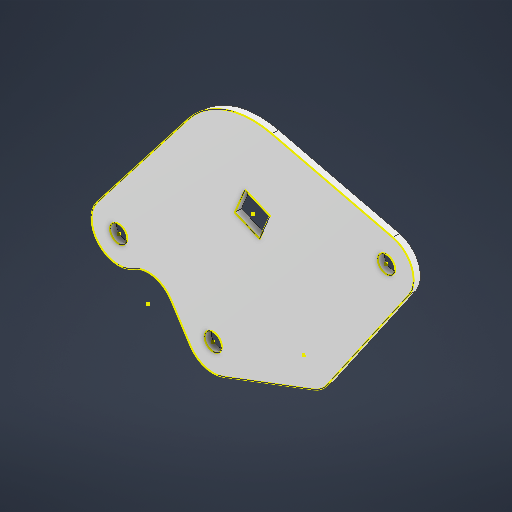
# Autodesk Inventor part: Rear Vertical Odom Pod
Saved by Autodesk Inventor 2025 (Build 290162010, 162A)
## iProperties
Created: 2024-10-31
Part Number: Rear Vertical Odom Pod
Material: Acetal Resin, White
Document SubType Name: Sheet Metal
Designer: blips
Density: 1.425 g/cm^3
Sheet Metal Rule: Default
Appearance: Smooth - White
Author: blips
Autodesk Inventor part; units mm, degrees
ref_plane "YZ Plane" through (0, 0, 0) normal (1, 0, 0) x (0, 1, 0)
ref_plane "XZ Plane" through (0, 0, 0) normal (0, 1, 0) x (-1, 0, 0)
ref_plane "XY Plane" through (0, 0, 0) normal (0, 0, 1) x (1, 0, 0)
sketch "Sketch1" plane through (0, 0, 0) normal (0, 0, 1) x (1, 0, 0)
  circle A0 centre (0, 0) radius 2.0955 construction
  circle A1 centre (31.2825, 19.6012) radius 7.2 construction
  circle A2 centre (43.3748, -2.7357) radius 2.15 construction
  circle A3 centre (31.2825, 19.6012) radius 31.75 construction
  circle A4 centre (43.3748, -2.7357) radius 2.032 construction
  line L0 (31.2825, 19.6012) -> (31.2825, -12.1488) construction
  circle A5 centre (31.2825, -12.1488) radius 2.032 construction
  line L1 (31.2825, 19.6012) -> (62.5502, 25.1146) construction
  line L2 (31.2825, 19.6012) -> (63.0325, 19.6012) construction
  circle A6 centre (62.5502, 25.1146) radius 2.032
  arc A7 (67.7804, 21.5135) -> (64.041, 31.2871) centre (62.5502, 25.1146) ccw
  circle A8 centre (0, 0) radius 2.032
  arc A9 (-5.017, 3.8926) -> (3.4439, -5.335) centre (0, 0) ccw
  arc A10 (45.62, -8.6755) -> (48.605, -6.3367) centre (43.3748, -2.7357) ccw
  circle A11 centre (22.0786, -10.7854) radius 2.032
  line L3 (48.605, -6.3367) -> (67.7804, 21.5135)
  arc A12 (35.755, 38.1188) -> (16.2316, 31.279) centre (31.2825, 19.6012) ccw
  line L4 (64.041, 31.2871) -> (35.755, 38.1188)
  line L5 (-5.017, 3.8926) -> (16.2316, 31.279)
  arc A13 (16.7437, -14.2294) -> (24.3239, -16.7253) centre (22.0786, -10.7854) ccw
  arc A14 (12.2228, -7.226) -> (3.4439, -5.335) centre (6.8878, -10.67) ccw
  line L6 (16.7437, -14.2294) -> (12.2228, -7.226)
  line L7 (45.9985, -8.5324) -> (24.3239, -16.7253)
  line L8 (27.7013, 17.6318) -> (32.3477, 15.7072)
  line L9 (27.7013, 17.6318) -> (27.7013, 17.6318)
  line L10 (32.3477, 15.7072) -> (27.7013, 17.6318)
  line L11 (32.3477, 15.7072) -> (32.3477, 15.7072)
  line L12 (33.1773, 16.0509) -> (35.1019, 20.6973)
  line L13 (33.1773, 16.0509) -> (33.1773, 16.0509)
  line L14 (35.1019, 20.6973) -> (33.1773, 16.0509)
  line L15 (35.1019, 20.6973) -> (35.1019, 20.6973)
  line L16 (34.7583, 21.5269) -> (30.1119, 23.4515)
  line L17 (34.7583, 21.5269) -> (34.7583, 21.5269)
  line L18 (30.1119, 23.4515) -> (34.7583, 21.5269)
  line L19 (30.1119, 23.4515) -> (30.1119, 23.4515)
  line L20 (29.2822, 23.1079) -> (27.3576, 18.4615)
  line L21 (29.2822, 23.1079) -> (29.2822, 23.1079)
  line L22 (27.3576, 18.4615) -> (29.2822, 23.1079)
  line L23 (27.3576, 18.4615) -> (27.3576, 18.4615)
  line L24 (35.1019, 20.6973) -> (35.3449, 21.2839)
  line L25 (34.7583, 21.5269) -> (35.3449, 21.2839)
  line L26 (33.1773, 16.0509) -> (32.9343, 15.4642)
  line L27 (32.3477, 15.7072) -> (32.9343, 15.4642)
  line L28 (29.2822, 23.1079) -> (29.5252, 23.6945)
  line L29 (30.1119, 23.4515) -> (29.5252, 23.6945)
  line L30 (27.3576, 18.4615) -> (27.1146, 17.8748)
  line L31 (27.7013, 17.6318) -> (27.1146, 17.8748)
  point P0 (0, 0)
extrude "Plate1" add sketch "Sketch1" along normal blind 1.5875
sketch "Sketch2" plane through (0, 0, 1.5875) normal (0, 0, 1) x (1, 0, 0)
  arc A0 (-5.017, 3.8926) -> (3.4439, -5.335) centre (0, 0) ccw projected
  line L0 (-5.017, 3.8926) -> (16.2316, 31.279) projected
  arc A1 (35.755, 38.1188) -> (16.2316, 31.279) centre (31.2825, 19.6012) ccw projected
  line L1 (35.755, 38.1188) -> (64.041, 31.2871) projected
  arc A2 (67.7804, 21.5135) -> (64.041, 31.2871) centre (62.5502, 25.1146) ccw projected
  line L2 (67.7804, 21.5135) -> (48.605, -6.3367) projected
  arc A3 (45.62, -8.6755) -> (48.605, -6.3367) centre (43.3748, -2.7357) ccw projected
  line L3 (45.62, -8.6755) -> (24.3239, -16.7253) projected
  arc A4 (16.7437, -14.2294) -> (24.3239, -16.7253) centre (22.0786, -10.7854) ccw projected
  line L4 (16.7437, -14.2294) -> (12.2228, -7.226) projected
  arc A5 (12.2228, -7.226) -> (3.4439, -5.335) centre (6.8878, -10.67) ccw projected
  circle A6 centre (0, 0) radius 2.032 projected
  circle A7 centre (22.0786, -10.7854) radius 2.032 projected
  circle A8 centre (62.5502, 25.1146) radius 2.032 projected
  line L5 (29.5252, 23.6945) -> (35.3449, 21.2839) projected
  line L6 (27.1146, 17.8748) -> (29.5252, 23.6945) projected
  line L7 (35.3449, 21.2839) -> (32.9343, 15.4642) projected
  line L8 (32.9343, 15.4642) -> (27.1146, 17.8748) projected
  point P0 (0, 0)
equation "\"d20\" = Thickness"
equation "\"BendRadius\" = Thickness"
equation "\"BendReliefWidth\" = Thickness"
equation "\"BendReliefDepth\" = 0.5 * Thickness"
equation "\"CornerReliefSize\" = 4 * Thickness"
equation "\"MinimumRemnant\" = 2 * Thickness"
equation "\"TransitionRadius\" = BendRadius"
equation "\"JacobiRadiusSize\" = BendRadius"
equation "\"GapSize\" = Thickness"
equation "\"Thickness\" = 1.5875"
body "Solid1"
